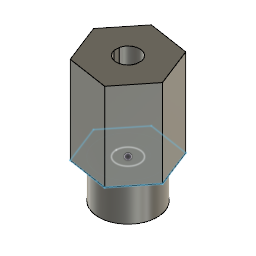
rc_car_tt_motor_adapter_12mm (Autodesk Fusion 360 design; units mm, degrees)
part number: 2026-02-21-14-01-04-154
Autodesk Fusion 360 part; units mm, degrees
sketch "Skizze1" plane through (0, 0, 0) normal (0, 0, 1) x (1, 0, 0)
  line L0 (1.95, -2.0094) -> (-1.95, 2.0094) construction
  line L1 (-1.95, 2.0094) -> (1.95, 2.0094)
  circle A0 centre (0, 0) radius 5
  line L2 (1.95, 2.0094) -> (1.95, -2.0094)
  line L3 (-1.95, -2.0094) -> (1.95, 2.0094) construction
  circle A1 centre (0, 0) radius 2.8
  line L4 (-1.95, -2.0094) -> (-1.95, 2.0094)
  line L5 (1.95, -2.0094) -> (-1.95, -2.0094)
  dimension "d1" = 5.6
  dimension "d2" = 10
  dimension "d3" = 3.9
  constraint coincident A0.centre A1.centre
  constraint horizontal L5
  constraint perpendicular L4 L5
  constraint parallel L1 L5
  constraint parallel L2 L4
  constraint coincident A0.centre L0
  constraint coincident A0.centre L3
  constraint coincident L0.end A1
  measures "d1" diameter of A1
  measures "d2" diameter of A0
  measures "d3" distance of L0.end L1.end
extrude "Extrusion1" add sketch "Skizze1" along normal blind 6.5 contours A1 L4 | L2 A1 | A0
sketch "Skizze2" plane through (0, 0, 6.5) normal (0, 0, 1) x (-1, 0, 0)
  arc A0 (-1.95, -2.0094) -> (1.95, -2.0094) centre (0, 0) ccw
  line L0 (-1.95, -2.0094) -> (-1.95, 2.0094)
  arc A1 (1.95, 2.0094) -> (-1.95, 2.0094) centre (0, 0) ccw
  line L1 (1.95, 2.0094) -> (1.95, -2.0094)
  circle A2 centre (0, 0) radius 5
  line L2 (-6.9634, 1.0605) -> (-4.4001, -5.5002)
  line L3 (-4.4001, -5.5002) -> (2.5632, -6.5607)
  line L4 (2.5632, -6.5607) -> (6.9634, -1.0605)
  line L5 (6.9634, -1.0605) -> (4.4001, 5.5002)
  line L6 (4.4001, 5.5002) -> (-2.5632, 6.5607)
  line L7 (-2.5632, 6.5607) -> (-6.9634, 1.0605)
  circle A3 centre (0, 0) radius 2
  dimension "d6" = 6.1
  dimension "d9" = 4
  constraint coincident A0.centre A1.centre
  measures "d6" distance of A0.centre L7
  measures "d9" diameter of A3
extrude "Extrusion2" add sketch "Skizze2" along normal blind 15 contours L0 A3 | L1 A3 | A2 | L2 L3 L4 L5 L6 L7
extrude "Extrusion3" add sketch "Skizze2" along normal blind 15 contours A0 L0 L1 A3 | L0 A1 L1 A3 | A2
